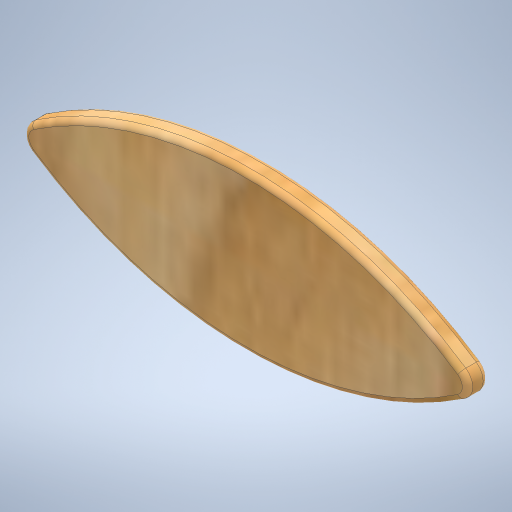
# Autodesk Inventor part: Lamello Biscuit S6
Saved by Autodesk Inventor 2024 (Build 280153000, 153)
## iProperties
Created: 2016-02-26
Part Number: Lamello Biscuit S6
Material: SW01
Description: Lamello
Document SubType Name: Modeling
Designer: S.Dereskevicius
Density: 0.721 g/cm^3
Appearance: SW01
Author: SauliusD
Autodesk Inventor part; units mm, degrees
ref_plane "YZ Plane" through (0, 0, 0) normal (1, 0, 0) x (0, 1, 0)
ref_plane "XZ Plane" through (0, 0, 0) normal (0, 1, 0) x (-1, 0, 0)
ref_plane "XY Plane" through (0, 0, 0) normal (0, 0, 1) x (1, 0, 0)
sketch "Sketch1" plane through (0, 0, 0) normal (0, 0, 1) x (1, 0, 0)
  line L0 (-63, 0) -> (63, 0) construction
  line L1 (45, 2) -> (-45, 2)
  line L2 (-45, 2) -> (-45, -2)
  line L3 (-45, -2) -> (45, -2)
  line L4 (45, -2) -> (45, 2)
  line L5 (45, -2) -> (-45, -2)
  line L6 (-45, -2) -> (-45, 2)
  line L7 (-45, 2) -> (45, 2)
  line L8 (45, 2) -> (45, -2)
  point P0 (0, 0)
  point P1 (0, 2)
  point P2 (-45, 0)
  dimension "d0" = 4
  dimension "d1" = 90
  constraints: 16 end point, 4 symmetric about line, 2 midpoint, 2 parallel, 1 horizontal, 1 perpendicular, 1 point on line, 1 vertical alignment
  measures "d0" distance of L1.end L2.end
  measures "d1" distance of L2.end L3.end
extrude "Groove Extrusion1" add sketch "Sketch1" along normal mid plane 40
sketch "Sketch2" plane through (0, 0, 0) normal (0, 1, 0) x (-1, 0, 0)
  line L0 (42.5, -15) -> (-42.5, -15) construction
  line L1 (-42.5, -15) -> (-42.5, 15) construction
  line L2 (-42.5, 15) -> (42.5, 15) construction
  line L3 (42.5, 15) -> (42.5, -15) construction
  line L4 (42.5, -15) -> (-42.5, 15) construction
  line L5 (-42.5, -15) -> (42.5, 15) construction
  arc A0 (41.1688, 2.493) -> (-41.1688, 2.493) centre (0, -59.0104) ccw
  arc A1 (-41.1688, -2.493) -> (41.1688, -2.493) centre (0, 59.0104) ccw
  arc A2 (41.1688, -2.493) -> (41.1688, 2.493) centre (39.5, 0) ccw
  arc A3 (-41.1688, 2.493) -> (-41.1688, -2.493) centre (-39.5, 0) ccw
  point P0 (0, 0)
  point P1 (0, 0)
  point P2 (0, 0)
  dimension "d7" = 3
  dimension "d8" = 85
  dimension "d9" = 30
  constraints: 12 end point, 8 point on circle, 8 tangent, 4 centre point, 4 midpoint, 2 parallel, 2 vertical alignment, 1 equal radius, 1 horizontal, 1 perpendicular
  measures "d7" radius of A3
  measures "d8" distance of L1.end L2.end
  measures "d9" distance of L2.end L0.start
extrude "Left Lamello Extrusion3" add sketch "Sketch2" along normal up to surface (4 mm away) from surface at -2 separate body
fillet "Left Lamello Fillet1" radius 1 8 edges at (42.5, -2, 0) (0, -2, -15) (-42.5, -2, 0) (0, -2, 15) (-42.5, 2, 0) (0, 2, -15) (42.5, 2, 0) (0, 2, 15)
equation "\"d0\" = Groove_T"
equation "\"d1\" = Groove_L"
equation "\"d3\" = 2 * Groove_W"
equation "\"d8\" = Lamello_L"
equation "\"d9\" = Lamello_W"
equation "\"d10\" = 2 * Groove_W"
equation "\"Groove_T\" = 4"
equation "\"Groove_L\" = 90"
equation "\"Lamello_W\" = 30"
equation "\"Lamello_L\" = 85"
equation "\"Lamello_T\" = 4"
equation "\"Groove_W\" = 20"
